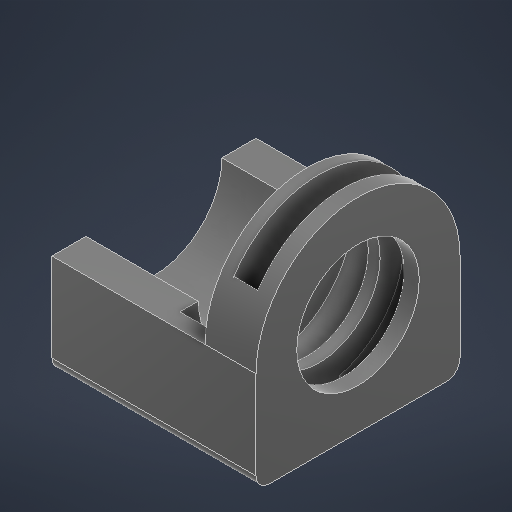
# Autodesk Inventor part: コリメータマウント
Saved by Autodesk Inventor 2026 (Build 300175050, 175E)
## iProperties
Created: 2025-07-11
Part Number: コリメータマウント
Material: 一般
Document SubType Name: Modeling
Designer: jin20
Density: 1 g/cm^3
Appearance: 滑らか - 黒
Author: jin20
Autodesk Inventor part; units mm, degrees
ref_plane "YZ Plane" through (0, 0, 0) normal (1, 0, 0) x (0, 1, 0)
ref_plane "XZ Plane" through (0, 0, 0) normal (0, 1, 0) x (-1, 0, 0)
ref_plane "XY Plane" through (0, 0, 0) normal (0, 0, 1) x (1, 0, 0)
sketch "スケッチ1" plane through (0, 0, 0) normal (1, 0, 0) x (0, 1, 0)
  line L0 (-15, 0) -> (-15, 15)
  line L1 (-15, 15) -> (0, 15)
  line L2 (-15, 0) -> (-15, -15)
  line L3 (-15, -15) -> (0, -15)
  arc A0 (0, -15) -> (0, 15) centre (0, 0) ccw
  dimension "d0" = 15
  dimension "d1" = 15
  dimension "d2" = 15
  dimension "d3" = 15
  dimension "d4" = 30
  constraints: 8 end point, 2 point on circle, 1 centre point, 1 coincident
  measures "d0" distance of L0.end L1.end
  measures "d1" distance of L0.start L0.end
  measures "d2" distance of L3.end L2.end
  measures "d3" distance of L2.end L2.start
  measures "d4" diameter of A0
extrude "押し出し1" add sketch "スケッチ1" along normal blind 30
sketch "スケッチ2" plane through (30, 0, 0) normal (1, 0, 0) x (0, 0, -1)
  circle A0 centre (0, 0) radius 9
  dimension "d7" = 18
  constraints: 1 centre point, 1 coincident
  measures "d7" diameter of A0
extrude "押し出し2" cut sketch "スケッチ2" against normal blind 7.5
sketch "スケッチ3" plane through (22.5, 0, 0) normal (1, 0, 0) x (0, 0, -1)
  circle A0 centre (0, 0) radius 12.7
  dimension "d10" = 25.4
  constraints: 1 centre point, 1 coincident
  measures "d10" diameter of A0
extrude "押し出し3" cut sketch "スケッチ3" against normal blind 6
sketch "スケッチ4" plane through (16.5, 0, 0) normal (1, 0, 0) x (0, 0, -1)
  circle A0 centre (0, 0) radius 10
  dimension "d13" = 20
  constraints: 1 centre point, 1 coincident
  measures "d13" diameter of A0
extrude "押し出し4" cut sketch "スケッチ4" against normal through all
sketch "スケッチ5" plane through (0, 0, 0) normal (-1, 0, 0) x (0, 0, 1)
  arc A0 (15, 0) -> (-15, 0) centre (0, 0) ccw
  line L0 (-15, 0) -> (15, 0)
  dimension "d16" = 30
  constraints: 2 end point, 2 point on circle, 1 centre point, 1 coincident, 1 horizontal
  measures "d16" diameter of A0
extrude "押し出し5" cut sketch "スケッチ5" against normal blind 22.5
sketch "スケッチ6" plane through (30, 0, 0) normal (1, 0, 0) x (0, 0, -1)
  arc A0 (-12.5, 0) -> (12.5, 0) centre (0, 0) ccw
  arc A1 (15, 0) -> (-15, 0) centre (0, 0) ccw projected
  line L0 (-12.5, 0) -> (12.5, 0)
  line L1 (12.5, 0) -> (12.5, 20)
  line L2 (12.5, 20) -> (-12.5, 20)
  line L3 (-12.5, 20) -> (-12.5, 0)
  point P0 (12.5, 8.2916)
  point P1 (-12.5, 8.2916)
  dimension "d19" = 25
  dimension "d20" = 25
  dimension "d21" = 20
  constraints: 8 end point, 2 parallel, 2 point on circle, 1 centre point, 1 coincident, 1 horizontal, 1 perpendicular
  measures "d19" diameter of A0
  measures "d20" distance of L2.end L1.end
  measures "d21" distance of L1.end L0.end
extrude "押し出し6" cut sketch "スケッチ6" against normal blind 5.75 contours L0 A0 | L3 A1 L1 L0
sketch "スケッチ7" plane through (30, 0, 0) normal (1, 0, 0) x (0, 0, -1)
  arc A0 (-12.5, 0) -> (12.5, 0) centre (0, 0) ccw
  arc A1 (15, 0) -> (-15, 0) centre (0, 0) ccw
  line L0 (-15, 0) -> (15, 0)
  dimension "d24" = 25
  dimension "d25" = 30
  constraints: 4 point on circle, 2 centre point, 2 coincident, 2 end point, 2 point on line, 1 horizontal
  measures "d24" diameter of A0
  measures "d25" diameter of A1
extrude "押し出し7" add sketch "スケッチ7" against normal blind 2.25
sketch "スケッチ8" plane through (30, 0, 0) normal (1, 0, 0) x (0, 0, -1)
  circle A0 centre (0, 0) radius 9
  dimension "d28" = 18
  constraints: 1 centre point, 1 coincident
  measures "d28" diameter of A0
extrude "押し出し8" cut sketch "スケッチ8" against normal through all
sketch "スケッチ9" plane through (0, -15, -15) normal (0, -1, 0) x (1, 0, 0)
  line L0 (0, 15) -> (26, 15) construction
  line L1 (27.75, 12) -> (24.25, 12)
  line L2 (24.25, 12) -> (24.25, 18)
  line L3 (24.25, 18) -> (27.75, 18)
  line L4 (27.75, 18) -> (27.75, 12)
  line L5 (27.75, 12) -> (24.25, 18) construction
  line L6 (24.25, 12) -> (27.75, 18) construction
  dimension "d31" = 26
  dimension "d32" = 3.5
  dimension "d33" = 6
  constraints: 14 end point, 2 horizontal, 2 midpoint, 2 parallel, 1 perpendicular
  measures "d31" distance of L0.start L0.end
  measures "d32" distance of L2.end L3.end
  measures "d33" distance of L1.end L2.end
extrude "押し出し9" cut sketch "スケッチ9" against normal through all
sketch "スケッチ10" plane through (0, -15, -15) normal (0, -1, 0) x (1, 0, 0)
  line L0 (0, 15) -> (12.5, 15) construction
  circle A0 centre (12.5, 15) radius 3
  dimension "d36" = 12.5
  dimension "d37" = 6
  constraints: 2 end point, 1 centre point, 1 coincident, 1 horizontal
  measures "d36" distance of L0.start L0.end
  measures "d37" diameter of A0
extrude "押し出し10" cut sketch "スケッチ10" against normal blind 5
thread "ねじ1" size "M6x1" class "6H" standard "ANSI Metric M Profile" full length
fillet "フィレット1" radius 2 2 edges at (15, -15, -15) (15, -15, 15)
